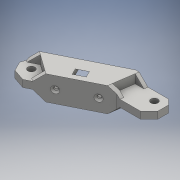
# Autodesk Inventor part: Support_GP2.Av
Saved by Autodesk Inventor 2016 (Build 200138000, 138)
## iProperties
Created: 2016-09-30
Part Number: Support_GP2.Av
Material: Générique
Document SubType Name: Modeling
Designer: LogOut
Density: 1 g/cm^3
Appearance: Par défaut
Author: LogOut
Autodesk Inventor part; units mm, degrees
ref_plane "YZ Plane" through (0, 0, 0) normal (1, 0, 0) x (0, 1, 0)
ref_plane "XZ Plane" through (0, 0, 0) normal (0, 1, 0) x (-1, 0, 0)
ref_plane "XY Plane" through (0, 0, 0) normal (0, 0, 1) x (1, 0, 0)
sketch "Esquisse1" plane through (0, 0, 0) normal (0, 0, 1) x (1, 0, 0)
  line L0 (156, 0) -> (156, 51.3475)
  line L1 (170, -60) -> (170, 60)
  line L2 (156, 0) -> (156, -52.5074)
  line L3 (-110, -100) -> (110, -100)
  line L4 (-54, 100) -> (-69, 100)
  line L5 (-78.695, 90) -> (-54, 90)
  line L6 (-156, 0) -> (-156, -52.5074)
  line L7 (-156, 0) -> (-156, 51.3475)
  line L8 (-170, 60) -> (-170, -60)
  line L9 (170, 60) -> (90, 100)
  line L10 (110, -100) -> (170, -60)
  line L11 (-170, -60) -> (-110, -100)
  line L12 (-90, 100) -> (-170, 60)
  line L13 (-156, 51.3475) -> (-78.695, 90)
  line L14 (-54, -90) -> (-54, 100)
  line L15 (-54, 100) -> (-81.0557, 100)
  line L16 (-81.0557, 100) -> (-166, 57.5279)
  line L17 (-166, 57.5279) -> (-166, 0)
  line L18 (-166, 0) -> (-166, -52.5074)
  line L19 (-54, 80) -> (-76.3344, 80)
  line L20 (-76.3344, 80) -> (-156, 40.1672)
  line L21 (-146, 45.1672) -> (-146, 0)
  line L22 (-146, 0) -> (-146, -52.5074)
  line L23 (-156, 51.3475) -> (-160.4721, 60.2918)
  line L24 (-156, 51.3475) -> (-151.5279, 42.4033)
  point P0 (54, -90)
  dimension "d9" = 14
  dimension "d10" = 14
  dimension "d11" = 10
  dimension "d14" = 108
  dimension "d15" = 10
  dimension "d16" = 10
  dimension "d17" = 56
  dimension "d18" = 56
  dimension "d19" = 14
  dimension "d20" = 14
  dimension "d21" = 14
  dimension "d22" = 14
  dimension "d25" = 10
  dimension "d26" = 10
  constraints: 50 end point, 7 point on line, 4 vertical, 2 perpendicular, 1 horizontal, 1 parallel, 3 other
  measures "d9" distance from line of L8 L6.start
  measures "d10" distance from line of L1 L0.start
  measures "d11" distance between parallel lines of L5 L4
  measures "d14" distance of point (54, -90) L14.start
  measures "d15" distance from line of L3 point (54, -90)
  measures "d16" distance from line of L3 L14.start
  measures "d17" horizontal distance of L11.end L14.start
  measures "d18" horizontal distance of L10.start point (54, -90)
  measures "d19" distance from line of L9 L0.end
  measures "d20" distance from line of L10 L2.end
  measures "d21" distance from line of L11 L6.end
  measures "d22" distance from line of L12 L7.end
  measures "d25" distance between parallel lines of L13 L16
  measures "d26" distance between parallel lines of L13 L20
extrude "Extrusion1" add sketch "Esquisse1" along normal blind 28 contours L14 L5 L13 L23 L16 L15 L4 | L14 L19 L20 L24 L13 L5
move faces "Déplacer1" translate (-10.7331, -5.3666, 0) faces at (-157.4907, 54.3289, 9.3333)
move faces "Déplacer2" translate (12, 0, 0) faces at (-54, 86.6667, 9.3333)
sketch "Esquisse2" plane through (0, 0, 28) normal (0, 0, 1) x (1, 0, 0)
  line L0 (-156, 51.3475) -> (-105.5104, 76.5923)
  line L1 (-171.2053, 54.9252) -> (-162.261, 37.0367) projected
  line L2 (-162.261, 37.0367) -> (-76.3344, 80) projected
  line L3 (-76.3344, 80) -> (-42, 80) projected
  line L4 (-42, 80) -> (-42, 100) projected
  line L5 (-42, 100) -> (-81.0557, 100) projected
  line L6 (-81.0557, 100) -> (-171.2053, 54.9252) projected
  line L7 (-42, 80) -> (-42, 100) projected
  line L8 (-42, 90) -> (-54, 90)
  dimension "d35" = 10
  dimension "d36" = 12
  dimension "d37" = 12
  constraints: 4 end point, 1 horizontal, 1 midpoint, 1 parallel
  measures "d35" distance between parallel lines of L6 L0
  measures "d36" distance from line of L1 L0.start
  measures "d37" distance of L8.start L8.end
hole "Perçage1" at (-156, 51.3475, 28) at (-54, 90, 28) direction (0, 0, -1) diameter 8 end through all
move faces "Déplacer3" translate (2.6833, -5.3666, 0) faces at (-133.6188, 51.3578, 9.3333)
move faces "Déplacer5" translate (0, -8, 0) faces at (-55.9453, 80, 18.6667)
move faces "Déplacer6" translate (-0.8944, 1.7889, 0) faces at (-111.1056, 84.9751, 9.3333)
sketch "Esquisse3" plane through (-172.0997, 56.7141, 28) normal (-0.4472136, 0.8944272, 0) x (0.8944272, 0.4472136, 0)
  line L0 (80.0902, 6) -> (32.0902, 6)
  line L1 (32.0902, 6) -> (32.0902, 22)
  line L2 (32.0902, 22) -> (80.0902, 22)
  line L3 (80.0902, 22) -> (80.0902, 6)
  line L4 (96.7902, 0) -> (0, 0) projected
  line L5 (96.7902, 28) -> (96.7902, 0) projected
  point P0 (128.5673, 28)
  dimension "d58" = 48
  dimension "d59" = 16
  dimension "d60" = 6
  dimension "d61" = 16.7
  constraints: 8 end point, 2 parallel, 1 horizontal, 1 perpendicular
  measures "d58" distance between parallel lines of L3 L1
  measures "d59" distance between parallel lines of L2 L0
  measures "d60" distance between parallel lines of L4 L0
  measures "d61" distance between parallel lines of L5 L3
extrude "Extrusion2" cut sketch "Esquisse3" against normal blind 24
sketch "Esquisse4" plane through (-161.3666, 35.2478, 28) normal (-0.4472136, 0.8944272, 0) x (0.8944272, 0.4472136, 0)
  line L0 (74.5902, 14) -> (37.5902, 14)
  line L1 (80.0902, 22) -> (80.0902, 6) projected
  line L2 (32.0902, 22) -> (80.0902, 22) projected
  point P0 (128.5673, 28)
  dimension "d64" = 37
  dimension "d65" = 5.5
  dimension "d66" = 8
  constraints: 2 end point, 1 horizontal
  measures "d64" distance of L0.start L0.end
  measures "d65" distance from line of L1 L0.start
  measures "d66" distance between parallel lines of L2 L0
hole "Perçage2" at (-94.651, 68.6056, 14) at (-127.7448, 52.0587, 14) direction (0.4472136, -0.8944272, 0) diameter 4 end through all
sketch "Esquisse5" plane through (-172.0997, 56.7141, 28) normal (-0.4472136, 0.8944272, 0) x (0.8944272, 0.4472136, 0)
  line L0 (96.7902, 6) -> (19.3902, 6)
  line L1 (19.3902, 6) -> (19.3902, 22)
  line L2 (19.3902, 22) -> (96.7902, 22)
  line L3 (96.7902, 22) -> (96.7902, 6)
  line L4 (80.0902, 6) -> (32.0902, 6) projected
  line L5 (32.0902, 22) -> (80.0902, 22) projected
  line L6 (96.7902, 28) -> (96.7902, 0) projected
  line L7 (80.0902, 22) -> (80.0902, 6) projected
  line L8 (32.0902, 6) -> (32.0902, 22) projected
  point P0 (128.5673, 28)
  dimension "d74" = 16.7
  dimension "d75" = 12.7
  constraints: 8 end point, 3 collinear, 2 parallel, 1 horizontal, 1 perpendicular
  measures "d74" distance between parallel lines of L3 L7
  measures "d75" distance between parallel lines of L8 L1
extrude "Extrusion3" cut sketch "Esquisse5" against normal blind 24 contours L0 L7 L2 L3 | L0 L1 L2 L8
chamfer "Chanfrein1" distance 24 distance2 16.7 1 edges at (-74.7938, 78.532, 14) measured on face at (-75.0175, 78.9792, 14)
chamfer "Chanfrein2" distance 24 distance2 12.7 1 edges at (-144.0225, 43.9176, 14) measured on face at (-144.2461, 44.3648, 14)
sketch "Esquisse6" plane through (0, 0, 28) normal (0, 0, 1) x (1, 0, 0)
  line L0 (-154.7565, 65.3857) -> (-132.6642, 49.599) projected
  line L1 (-132.6642, 49.599) -> (-154.7565, 65.3857) projected
  line L2 (-85.5279, 100) -> (-89.7317, 71.0653) projected
  line L3 (-89.7317, 71.0653) -> (-85.5279, 100) projected
  line L4 (-81.4859, 100) -> (-86.0737, 68.4221)
  line L5 (-158.8043, 63.3618) -> (-133.0299, 44.944)
  circle A0 centre (-156, 51.3475) radius 4 projected
  circle A1 centre (-54, 90) radius 4 projected
  line L6 (-172.0997, 56.7141) -> (-159.5777, 31.6701) projected
  line L7 (-159.5777, 31.6701) -> (-78.918, 72) projected
  line L8 (-78.918, 72) -> (-42, 72) projected
  line L9 (-42, 72) -> (-42, 100) projected
  line L10 (-42, 100) -> (-85.5279, 100) projected
  line L11 (-85.5279, 100) -> (-172.0997, 56.7141) projected
  point P0 (0, 0)
  dimension "d84" = 4
  dimension "d85" = 4
  constraints: 4 end point, 4 point on line, 2 parallel
  measures "d84" distance between parallel lines of L2 L4
  measures "d85" distance between parallel lines of L0 L5
extrude "Extrusion4" cut sketch "Esquisse6" against normal blind 10 contours L10 L9 L8 L7 L4 | L7 L6 L11 L5
ref_plane "Plan de construction1" through (-89.7317, 71.0653, 14) normal (0, 0, 1) x (0.9896102, -0.1437764, 0)
mirror "Symétrie1" about plane through (-89.7317, 71.0653, 14) normal (0, 0, 1) of "Extrusion4"
chamfer "Chanfrein3" distance 10 angle 45 4 edges at (-83.7798, 84.2111, 18) (-83.7798, 84.2111, 10) (-145.9171, 54.1529, 10) (-145.9171, 54.1529, 18)
sketch "Esquisse7" plane through (0, 0, 28) normal (0, 0, 1) x (1, 0, 0)
  line L0 (-78.918, 72) -> (-75.4489, 72) projected
  line L1 (-86.0737, 68.4221) -> (-78.918, 72) projected
  line L2 (-71.3809, 100) -> (-81.4859, 100) projected
  line L3 (-143.1492, 39.8844) -> (-133.0299, 44.944) projected
  line L4 (-158.8043, 63.3618) -> (-168.9236, 58.3021) projected
  line L5 (-85.3731, 73.2446) -> (-79.8622, 76)
  line L6 (-79.8622, 76) -> (-74.8677, 76)
  line L7 (-71.962, 96) -> (-82.067, 96)
  line L8 (-146.8313, 42.5155) -> (-136.7119, 47.5752)
  line L9 (-155.1222, 60.7307) -> (-165.2416, 55.671)
  line L10 (-75.4489, 72) -> (-71.3809, 100) projected
  line L11 (-86.0737, 68.4221) -> (-81.4859, 100) projected
  line L12 (-158.8043, 63.3618) -> (-133.0299, 44.944) projected
  line L13 (-154.1954, 47.7777) -> (-143.1492, 39.8844) projected
  line L14 (-168.9236, 58.3021) -> (-159.9619, 51.8983) projected
  arc A0 (-154.1954, 47.7777) -> (-159.9619, 51.8983) centre (-156, 51.3475) ccw projected
  point P0 (0, 0)
  dimension "d92" = 4
  dimension "d93" = 4
  dimension "d94" = 4
  dimension "d95" = 4
  constraints: 10 end point, 8 point on line, 3 parallel
  measures "d92" distance between parallel lines of L1 L5
  measures "d93" distance between parallel lines of L2 L7
  measures "d94" distance between parallel lines of L3 L8
  measures "d95" distance between parallel lines of L4 L9
extrude "Extrusion5" cut sketch "Esquisse7" against normal blind 10 contours L6 L5 L11 L7 L10 | L13 A0 L14 L9 L12 L8
mirror "Symétrie2" about plane through (-89.7317, 71.0653, 14) normal (0, 0, 1) of "Extrusion5"
chamfer "Chanfrein5" distance 6 angle 45 2 edges at (-42, 100, 14) (-172.0997, 56.7141, 14)
chamfer "Chanfrein6" distance 10 angle 45 2 edges at (-42, 72, 14) (-159.5777, 31.6701, 14)
sketch "Esquisse8" plane through (0, 0, 28) normal (0, 0, 1) x (1, 0, 0)
  line L0 (-110.3035, 71.9597) -> (-121.0366, 66.5931)
  line L1 (-121.0366, 66.5931) -> (-117.4589, 59.4377)
  line L2 (-117.4589, 59.4377) -> (-106.7258, 64.8043)
  line L3 (-106.7258, 64.8043) -> (-110.3035, 71.9597)
  line L4 (-133.0299, 44.944) -> (-86.0737, 68.4221) projected
  line L5 (-132.6642, 49.599) -> (-89.7317, 71.0653) projected
  point P0 (0, 0)
  dimension "d107" = 6
  dimension "d108" = 8
  dimension "d109" = 12
  dimension "d110" = 18
  dimension "d111" = 18
  constraints: 8 end point, 3 parallel, 1 perpendicular
  measures "d107" distance between parallel lines of L4 L2
  measures "d108" distance between parallel lines of L2 L0
  measures "d109" distance between parallel lines of L3 L1
  measures "d110" distance from line of L5.start L1
  measures "d111" distance from line of L5.end L3
extrude "Extrusion6" cut sketch "Esquisse8" against normal blind 10
chamfer "Chanfrein7" distance 8 distance2 6 1 edges at (-115.6701, 69.2764, 22) measured on face at (-115.8937, 69.7236, 22)
chamfer "Chanfrein8" distance 2 angle 45 4 edges at (-120.1422, 82.6928, 22) (-120.1422, 82.6928, 6) (-125.956, 48.481, 12) (-92.8622, 65.0279, 12)
